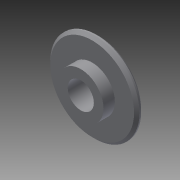
# Autodesk Inventor part: Sprocket Large
Saved by Autodesk Inventor 2015 (Build 190159000, 159)
## iProperties
Created: 2015-01-11
Part Number: Sprocket Large
Material: Generic
Document SubType Name: Modeling
Designer: chapale16
Density: 1 g/cm^3
Appearance: Default
Author: chapale16
Autodesk Inventor part; units mm, degrees
ref_plane "YZ Plane" through (0, 0, 0) normal (1, 0, 0) x (0, 1, 0)
ref_plane "XZ Plane" through (0, 0, 0) normal (0, 1, 0) x (-1, 0, 0)
ref_plane "XY Plane" through (0, 0, 0) normal (0, 0, 1) x (1, 0, 0)
sketch "Sketch1" plane through (0, 0, 0) normal (0, 0, 1) x (1, 0, 0)
  circle A0 centre (0, 0) radius 24.9555
  circle A1 centre (0, 0) radius 7.3025
  dimension "d0" = 49.911
  dimension "d2" = 14.605
  constraints: 2 centre point, 1 coincident
  measures "d0" diameter of A0
  measures "d2" diameter of A1
extrude "Extrusion1" add sketch "Sketch1" along normal blind 3.937
sketch "Sketch2" plane through (0, 0, 3.937) normal (0, 0, 1) x (1, 0, 0)
  circle A0 centre (0, 0) radius 7.3025
  circle A1 centre (0, 0) radius 12.7
  dimension "d5" = 25.4
  constraints: 2 centre point, 2 coincident
  measures "d5" diameter of A1
extrude "Extrusion2" add sketch "Sketch2" along normal blind 6.35
chamfer "Chamfer1" distance 1.524 angle 45 1 edges at (-24.9555, 0, 3.937)
chamfer "Chamfer2" distance 1.524 angle 45 1 edges at (-24.9555, 0, 0)
body "Solid1"
